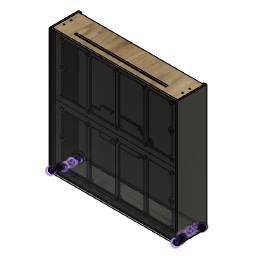
LEDMatrixCAD (Autodesk Fusion 360 design; units mm, degrees)
Autodesk Fusion 360 part; units mm, degrees
note: some values were not read from the file. Set by a fixed rule: which sketch regions a step uses.
sketch "PanelMount" plane through (0, 0, 0) normal (0, 1, 0) x (1, 0, 0)
  line L0 (0, 0) -> (256, 0)
  line L1 (256, 0) -> (256, -128)
  line L2 (256, -128) -> (0, -128)
  line L3 (0, -128) -> (0, 0)
  line L4 (128, -128) -> (128, 0) construction
  circle A0 centre (128, -116.25) radius 2.325
  circle A1 centre (128, -116.25) radius 6.975
  line L5 (0, -64) -> (256, -64) construction
  circle A2 centre (188, -116.25) radius 2.325
  circle A3 centre (188, -116.25) radius 6.975
  circle A4 centre (244, -116.25) radius 6.975
  circle A5 centre (244, -116.25) radius 2.325
  line L6 (244, -128) -> (244, 0) construction
  circle A6 centre (244, -64) radius 6.975
  circle A7 centre (244, -64) radius 2.325
  circle A8 centre (68, -116.25) radius 6.975
  circle A9 centre (68, -116.25) radius 2.325
  circle A10 centre (12, -116.25) radius 6.975
  circle A11 centre (12, -116.25) radius 2.325
  circle A12 centre (12, -64) radius 6.975
  circle A13 centre (12, -64) radius 2.325
  circle A14 centre (12, -11.75) radius 2.325
  circle A15 centre (12, -11.75) radius 6.975
  circle A16 centre (68, -11.75) radius 2.325
  circle A17 centre (68, -11.75) radius 6.975
  circle A18 centre (128, -11.75) radius 2.325
  circle A19 centre (128, -11.75) radius 6.975
  circle A20 centre (188, -11.75) radius 2.325
  circle A21 centre (188, -11.75) radius 6.975
  circle A22 centre (244, -11.75) radius 2.325
  circle A23 centre (244, -11.75) radius 6.975
  line L7 (12, -116.25) -> (244, -116.25)
  line L8 (244, -116.25) -> (244, -11.75)
  line L9 (244, -11.75) -> (12, -11.75)
  line L10 (12, -11.75) -> (12, -116.25)
  line L11 (0, -128) -> (-3, -128)
  line L12 (-3, -128) -> (-3, 0)
  line L13 (-3, 0) -> (0, 0)
  line L14 (256, -128) -> (259, -128)
  line L15 (259, -128) -> (259, 0)
  line L16 (259, 0) -> (256, 0)
  line L17 (65, -116.25) -> (65, -11.75)
  line L18 (71, -11.75) -> (71, -116.25)
  line L19 (68, -116.25) -> (68, -11.75) construction
  line L20 (125, -116.25) -> (125, -11.75)
  line L21 (131, -11.75) -> (131, -116.25)
  line L22 (131, -87.1298) -> (125, -87.1298) construction
  line L23 (65, -82.2396) -> (71, -82.2396) construction
  line L24 (185, -11.75) -> (185, -116.25)
  line L25 (191, -116.25) -> (191, -11.75)
  dimension "d301" = 4.65
  dimension "d302" = 4.65
  dimension "d305" = 60
  dimension "d306" = 116
  dimension "d308" = 256
  dimension "d309" = 128
  dimension "d310" = 11.75
  dimension "d348" = 3
  dimension "d429" = 6
  constraint horizontal L0
  constraint vertical L1
  constraint horizontal L2
  constraint vertical L3
  constraint coincident L0.start L3.end
  constraint midpoint L2 L4.start
  constraint midpoint L0 L4.end
  constraint coincident L4 A0.centre
  constraint concentric A0 A1
  constraint coincident L3 L5.start
  constraint coincident L1 L5.end
  constraint perpendicular L1 L5
  constraint midpoint L3 L5.start
  constraint concentric A2 A3
  constraint equal A1 A3
  constraint equal A0 A2
  constraint concentric A4 A5
  constraint equal A1 A4
  constraint equal A0 A5
  constraint coincident L2 L6.start
  constraint coincident L0 L6.end
  constraint perpendicular L0 L6
  constraint coincident A4.centre L6
  constraint concentric A6 A7
  constraint coincident L5 A6.centre
  constraint coincident L6 A6.centre
  constraint equal A1 A6
  constraint equal A0 A7
  constraint symmetric L4 A2 A9
  constraint symmetric L4 A3 A8
  constraint symmetric L4 A4 A10
  constraint symmetric L4 A5 A11
  constraint symmetric L4 A6 A12
  constraint symmetric L4 A7 A13
  constraint symmetric A0 L5 A18
  constraint symmetric A1 L5 A19
  constraint symmetric L5 A2 A20
  constraint symmetric L5 A3 A21
  constraint symmetric L5 A4 A23
  constraint symmetric L5 A5 A22
  constraint symmetric L5 A8 A17
  constraint symmetric L5 A9 A16
  constraint symmetric L5 A10 A15
  constraint symmetric L5 A11 A14
  constraint horizontal L7
  constraint vertical L8
  constraint horizontal L9
  constraint vertical L10
  constraint coincident A22.centre A23.centre
  constraint coincident A10.centre A11.centre
  constraint coincident A0.centre L7
  constraint coincident A2.centre L7
  constraint perpendicular L3 L11
  constraint perpendicular L11 L12
  constraint perpendicular L3 L13
  constraint perpendicular L1 L14
  constraint perpendicular L14 L15
  constraint perpendicular L1 L16
  constraint equal L11 L14
  constraint coincident L7 L17.start
  constraint coincident L9 L17.end
  constraint perpendicular L9 L17
  constraint coincident L9 L18.start
  constraint coincident L7 L18.end
  constraint perpendicular L7 L18
  constraint coincident A8.centre A9.centre
  constraint coincident A16.centre A17.centre
  constraint coincident L7 L20.start
  constraint coincident L9 L20.end
  constraint perpendicular L9 L20
  constraint coincident L9 L21.start
  constraint coincident L7 L21.end
  constraint perpendicular L7 L21
  constraint symmetric L4 L20 L21
  constraint coincident L21 L22.start
  constraint coincident L20 L22.end
  constraint perpendicular L20 L22
  constraint coincident L17 L23.start
  constraint coincident L18 L23.end
  constraint perpendicular L18 L23
  constraint equal L22 L23
  constraint symmetric L4 L17.start L25.start
  constraint symmetric L4 L17.end L25.end
  constraint symmetric L4 L18.start L24.start
  constraint symmetric L4 L18.end L24.end
  measures "d301" diameter of A0
  measures "d302" distance of A0 A1
  measures "d305" distance of A0.centre A2.centre
  measures "d306" distance of A0.centre A4.centre
  measures "d308" distance of L1.end L2.end
  measures "d309" distance of L0.start L2.end
  measures "d310" distance of L2 L7
  measures "d348" distance of L2.end L11.end
  measures "d429" distance of L17 L18
extrude "Extrude3" add sketch "PanelMount" against normal blind 3 contours L0 L1 L2 L3 | L3 L11 L12 L13 | L1 L14 L15 L16 | A0 A1 L7 | A0 A1 L7 L20 L21 | A1 L7 L21 | A1 L7 L20 | A1 A19 L20 L21 | A2 A3 L7 | A3 L7 L24 | A19 L9 L21 | A18 A19 L9 L20 L21 | A8 L7 L18 | A8 A9 L7 | A19 L9 L20 | A3 A21 L24 L25 | A2 A3 L7 L24 L25 | A3 L7 L25 | A18 A19 L9 | A8 A9 L7 L17 L18 | A8 A17 L17 L18 | A8 L7 L17 | A20 A21 L9 L24 L25 | A21 L9 L24 | A4 A5 L7 L8 | A4 A5 L7 L8 | A20 A21 L9 | A17 L9 L18 | A16 A17 L9 L17 L18 | A10 A11 L7 L10 | A10 A11 L7 L10 | A16 A17 L9 | A21 L9 L25 | A17 L9 L17 | A6 A7 L8 | A6 A7 L8 | A22 A23 L8 L9 | A22 A23 L8 L9 | A12 A13 L10 | A12 A13 L10 | A14 A15 L9 L10 | A14 A15 L9 L10 makes body 1
ref_plane "WorkPlane2" through (128, -1.5, 64) normal (1, 0, 0) x (0, 0, 1)
fillet "Fillet1" radius 1.5 12 edges at (9.8323, -3, 117.0908) (65.8323, -3, 117.0908) (125.8323, -3, 117.0908) (185.8323, -3, 117.0908) (241.8323, -3, 117.0908) (241.8323, -3, 64.8408) (241.8323, -3, 12.5908) (185.8323, -3, 12.5908) (125.8323, -3, 12.5908) (65.8323, -3, 12.5908) (9.8323, -3, 12.5908) (9.8323, -3, 64.8408) on bodies 1
pattern_linear "R-Pattern2" count 1 spacing 256 along (1, 0, 0) count 2 spacing 128 along (0, 0, 1) of bodies 1 makes body 2
sketch "Bracket" plane through (0, 0, 0) normal (0, 0, 1) x (1, 0, 0)
  line L0 (-6.65, -10.875) -> (-6.65, 51.475)
  line L1 (-6.65, 51.475) -> (-0.65, 51.475)
  line L2 (-0.65, -3.5) -> (-3.65, -3.5)
  line L3 (-3.65, -3.5) -> (-3.65, 0.5)
  line L4 (-3.65, 0.5) -> (-0.65, 0.5)
  line L5 (-0.65, 0) -> (-0.65, -3.5)
  line L6 (-0.65, 0.5) -> (-0.65, 0)
  line L7 (-0.65, -3.5) -> (-0.65, -7.5)
  line L8 (-0.65, -3) -> (-0.65, -3.5)
  line L9 (-0.65, 51.475) -> (-0.65, 0.5)
  line L10 (-0.65, 0) -> (-0.65, -3)
  line L11 (128, 11.7514) -> (128, -14.585) construction
  line L12 (-0.65, -7.5) -> (-3.65, -7.5)
  line L13 (-3.65, -7.5) -> (-3.65, -10.875)
  line L14 (-3.65, 0.5) -> (-3.65, 43.5)
  line L15 (-3.65, -3.5) -> (-3.65, -7.5)
  line L16 (-3, 0) -> (259, 0)
  line L17 (259, 0) -> (259, -3)
  line L18 (259, -3) -> (-3, -3)
  line L19 (-3, -3) -> (-3, 0)
  line L20 (-3.65, 43.5) -> (-0.65, 43.5)
  line L21 (-3.65, 43.5) -> (-3.65, 47.975)
  line L22 (-3.65, 47.975) -> (-0.65, 47.975)
  line L23 (-0.65, 38.5) -> (7.35, 38.5)
  line L24 (7.35, 38.5) -> (7.35, 43.5)
  line L25 (7.35, 43.5) -> (-0.65, 43.5)
  line L26 (-6.65, 18) -> (7.35, 18) construction
  line L27 (-0.65, 6.5) -> (7.35, 6.5)
  line L28 (7.35, 6.5) -> (7.35, 29.5)
  line L29 (7.35, 29.5) -> (-0.65, 29.5)
  circle A0 centre (3.35, 25.5) radius 1.5
  line L30 (3.35, 6.5) -> (3.35, 29.5) construction
  circle A1 centre (3.35, 10.5) radius 1.5
  line L31 (-3.65, -10.875) -> (-6.65, -10.875)
  line L32 (7.35, 43.5) -> (20, 43.5) construction
  line L33 (20, 43.5) -> (20, -7.5) construction
  line L34 (20, -7.5) -> (-0.65, -7.5) construction
  line L35 (20, 18) -> (7.35, 18) construction
  point P0 (128, 0)
  point P1 (128, 0)
  dimension "d334" = 4
  dimension "d335" = 3.375
  dimension "d349" = 0.65
  dimension "d350" = 0.5
  dimension "d351" = 0.5
  dimension "d353" = 3
  dimension "d354" = 3
  dimension "d356" = 43
  dimension "d359" = 4.475
  dimension "d360" = 3.5
  dimension "d361" = 8
  dimension "d362" = 5
  dimension "d366" = 8
  dimension "d376" = 3
  dimension "d379" = 4
  dimension "d452" = 23
  constraint vertical L9
  constraint perpendicular L1 L9
  constraint coincident L5.start L9
  constraint horizontal L2
  constraint vertical L3
  constraint horizontal L4
  constraint vertical L5
  constraint coincident L2.start L9
  constraint equal L6 L8
  constraint collinear L9 L10
  constraint perpendicular L12 L13
  constraint equal L2 L12
  constraint coincident L11 P1
  constraint coincident L9 L20.end
  constraint perpendicular L9 L20
  constraint perpendicular L20 L21
  constraint coincident L9 L22.end
  constraint perpendicular L9 L22
  constraint coincident L9 L23.start
  constraint perpendicular L9 L23
  constraint perpendicular L20 L24
  constraint perpendicular L9 L25
  constraint perpendicular L9 L26
  constraint coincident L9 L27.start
  constraint perpendicular L9 L27
  constraint perpendicular L27 L28
  constraint coincident L9 L29.end
  constraint perpendicular L9 L29
  constraint midpoint L28 L26.end
  constraint midpoint L27 L30.start
  constraint midpoint L29 L30.end
  constraint coincident A0.centre L30
  constraint symmetric L26 A0 A1
  constraint perpendicular L0 L31
  constraint coincident L0 L26.start
  constraint perpendicular L7 L12
  constraint perpendicular L24 L32
  constraint perpendicular L12 L33
  constraint perpendicular L7 L34
  constraint midpoint L33 L35.start
  constraint perpendicular L33 L35
  measures "d334" distance of L2 L12
  measures "d335" distance of L12.end L13.end
  measures "d349" distance of L3 L19
  measures "d350" distance of L2 L18
  measures "d351" distance of L4 L16
  measures "d353" distance of L9 L14
  measures "d354" distance of L0 L3
  measures "d356" distance of L4 L20
  measures "d359" distance of L20 L22
  measures "d360" distance of L1 L22
  measures "d361" distance of L9 L24
  measures "d362" distance of L23 L25
  measures "d366" distance of L27.start L27.end
  measures "d376" diameter of A0
  measures "d379" distance of L29 A0.centre
  measures "d452" distance of L27.end L28.end
extrude "Extrude4" add sketch "Bracket" along normal blind 256 separate body contours L0 L1 L3 L9 L13 L14 L15 L21 L22 L31 | L2 L7 L12 L15 | L4 L9 L14 L20 makes body 3
extrude "Extrude5" add sketch "Bracket" along normal blind 3.175 from surface at 256 contours L0 L1 L3 L9 L13 L14 L15 L21 L22 L31 bodies 3
extrude "Extrude6" add sketch "Bracket" against normal blind 3.175 contours L0 L1 L3 L9 L13 L14 L15 L21 L22 L31 bodies 3
extrude "Extrude7" add sketch "Bracket" along normal blind 8 contours L9 L23 L24 L25 bodies 3
extrude "Extrude8" add sketch "Bracket" along normal blind 3 contours L9 L27 L28 L29 bodies 3
sketch "MountTabHole" plane through (0, 43.5, 0) normal (0, 1, 0) x (-1, 0, 0)
  line L0 (-7.35, 0) -> (3.65, 0)
  line L1 (3.65, 0) -> (3.65, 256)
  line L2 (3.65, 256) -> (0.65, 256)
  line L3 (0.65, 256) -> (0.65, 8)
  line L4 (0.65, 8) -> (-7.35, 8)
  line L5 (-7.35, 8) -> (-7.35, 0)
  line L6 (0.65, 8) -> (0.65, 0)
  line L7 (-7.35, 8) -> (0.65, 0) construction
  line L8 (-7.35, 0) -> (0.65, 8) construction
  circle A0 centre (-3.35, 4) radius 1.5
  dimension "d383" = 3
  constraint coincident L3.end L4.start
  constraint coincident L0 L6.end
  constraint perpendicular L0 L6
  constraint coincident L4.end L5.start
  constraint coincident L0.start L5.end
  constraint midpoint L7 A0.centre
  measures "d383" diameter of A0
extrude "Extrude9" cut sketch "MountTabHole" against normal up to surface (5 mm away) contours A0 bodies 3
ref_plane "WorkPlane3" through (-3.65, 20.3, 128) normal (0, 0, 1) x (1, 0, 0)
mirror "Mirror5" about plane through (-3.65, 20.3, 128) normal (0, 0, 1) of "Extrude7", "Extrude8", "Extrude9"
mirror "Mirror2" about plane through (128, -1.5, 64) normal (1, 0, 0) of bodies 3 makes body 4
sketch "PiMount" plane through (0, 0, 0) normal (0, 1, 0) x (1, 0, 0)
  line L0 (128, -128) -> (128, 0)
  line L1 (166.5, -156.5) -> (89.5, -156.5)
  line L2 (85.5, -152.5) -> (85.5, -103.5)
  line L3 (89.5, -99.5) -> (166.5, -99.5)
  line L4 (170.5, -103.5) -> (170.5, -152.5)
  line L5 (166.5, -152.5) -> (108.5, -152.5) construction
  line L6 (108.5, -152.5) -> (108.5, -103.5) construction
  line L7 (108.5, -103.5) -> (166.5, -103.5) construction
  line L8 (166.5, -103.5) -> (166.5, -152.5) construction
  circle A0 centre (166.5, -152.5) radius 1.7
  circle A1 centre (108.5, -152.5) radius 1.7
  circle A2 centre (166.5, -103.5) radius 1.7
  circle A3 centre (108.5, -103.5) radius 1.7
  line L9 (166.5, -152.5) -> (166.5, -156.5) construction
  line L10 (166.5, -103.5) -> (166.5, -99.5) construction
  arc A4 (166.5, -156.5) -> (170.5, -152.5) centre (166.5, -152.5) ccw
  arc A5 (170.5, -103.5) -> (166.5, -99.5) centre (166.5, -103.5) ccw
  arc A6 (89.5, -99.5) -> (85.5, -103.5) centre (89.5, -103.5) ccw
  arc A7 (85.5, -152.5) -> (89.5, -156.5) centre (89.5, -152.5) ccw
  line L11 (128, -156.5) -> (128, -99.5) construction
  circle A8 centre (188, -116.25) radius 2.325
  circle A9 centre (188, -139.75) radius 2.325
  circle A10 centre (68, -139.75) radius 2.325
  circle A11 centre (68, -116.25) radius 2.325
  line L12 (172.5, -145.75) -> (190, -145.75)
  line L13 (194, -141.75) -> (194, -114.25)
  line L14 (190, -110.25) -> (172.5, -110.25)
  line L15 (256, -128) -> (0, -128)
  line L16 (188, -139.75) -> (188, -145.75) construction
  line L17 (188, -139.75) -> (194, -139.75) construction
  arc A12 (190, -145.75) -> (194, -141.75) centre (190, -141.75) ccw
  arc A13 (194, -114.25) -> (190, -110.25) centre (190, -114.25) ccw
  arc A14 (172.5, -145.75) -> (170.5, -147.75) centre (172.5, -147.75) ccw
  arc A15 (170.5, -108.25) -> (172.5, -110.25) centre (172.5, -108.25) ccw
  arc A16 (83.5, -110.25) -> (85.5, -108.25) centre (83.5, -108.25) ccw
  line L18 (66, -110.25) -> (83.5, -110.25)
  arc A17 (66, -110.25) -> (62, -114.25) centre (66, -114.25) ccw
  line L19 (62, -141.75) -> (62, -114.25)
  arc A18 (62, -141.75) -> (66, -145.75) centre (66, -141.75) ccw
  line L20 (83.5, -145.75) -> (66, -145.75)
  arc A19 (85.5, -147.75) -> (83.5, -145.75) centre (83.5, -147.75) ccw
  circle A20 centre (188, -139.75) radius 1.575
  circle A21 centre (188, -116.25) radius 1.575
  circle A22 centre (68, -139.75) radius 1.575
  circle A23 centre (68, -116.25) radius 1.575
  circle A24 centre (188, -139.75) radius 3.5
  point P0 (170.5, -156.5)
  point P1 (85.5, -156.5)
  dimension "d406" = 85
  dimension "d408" = 3.4
  dimension "d409" = 4
  dimension "d410" = 4
  dimension "d411" = 49
  dimension "d412" = 58
  dimension "d413" = 4
  dimension "d414" = 6
  dimension "d415" = 4
  dimension "d416" = 4
  dimension "d417" = 4
  dimension "d426" = 3.15
  dimension "d428" = 3.5
  constraint horizontal L1
  constraint vertical L2
  constraint horizontal L3
  constraint vertical L4
  constraint horizontal L5
  constraint vertical L6
  constraint horizontal L7
  constraint vertical L8
  constraint coincident L5.start L8.end
  constraint coincident L5.end L6.start
  constraint coincident L7.end L8.start
  constraint coincident L6.end L7.start
  constraint equal A0 A1
  constraint equal A0 A2
  constraint equal A0 A3
  constraint coincident L1 L9.end
  constraint perpendicular L1 L9
  constraint coincident L3 L10.end
  constraint perpendicular L3 L10
  constraint equal L9 L10
  constraint coincident P0 L1
  constraint coincident P0 L4
  constraint tangent L1 A4
  constraint tangent L4 A4
  constraint tangent L3 A5
  constraint tangent L4 A5
  constraint equal A4 A5
  constraint tangent L2 A6
  constraint tangent L3 A6
  constraint equal A4 A6
  constraint coincident P1 L1
  constraint coincident P1 L2
  constraint tangent L1 A7
  constraint tangent L2 A7
  constraint equal A4 A7
  constraint midpoint L1 L11.start
  constraint midpoint L3 L11.end
  constraint coincident L0 L11.end
  constraint perpendicular L4 L12
  constraint perpendicular L12 L13
  constraint perpendicular L4 L14
  constraint symmetric L12 L14 L15
  constraint coincident A9.centre L16.start
  constraint coincident L12 L16.end
  constraint perpendicular L12 L16
  constraint coincident L13 L17.end
  constraint perpendicular L13 L17
  constraint equal L16 L17
  constraint tangent L12 A12
  constraint tangent L13 A12
  constraint tangent L13 A13
  constraint tangent L14 A13
  constraint equal A12 A13
  constraint tangent L4 A14
  constraint tangent L12 A14
  constraint coincident L4 A14.end
  constraint tangent L14 A15
  constraint tangent L4 A15
  constraint coincident L4 A15.start
  constraint symmetric L11 L12.end A18.end
  constraint symmetric L11 L13.start L19.start
  constraint symmetric L11 A12 A18
  constraint symmetric L11 L13.end A17.end
  constraint symmetric L11 L14.start L18.start
  constraint symmetric L11 A13 A17
  constraint symmetric L11 A14.end A19.start
  constraint symmetric L11 L12.start L20.start
  constraint symmetric L11 A14 A19
  constraint symmetric L11 L14.end A16.start
  constraint symmetric L11 A15.start A16.end
  constraint symmetric L11 A15 A16
  constraint symmetric L1 L3 L15
  constraint concentric A9 A20
  constraint concentric A8 A21
  constraint equal A20 A21
  constraint symmetric L11 A20 A22
  constraint symmetric L11 A21 A23
  constraint concentric A9 A24
  measures "d406" distance of P0 P1
  measures "d408" diameter of A0
  measures "d409" distance of L1 L5.start
  measures "d410" distance of L4 L5.start
  measures "d411" distance of L5.start L7.end
  measures "d412" distance of L5.start L5.end
  measures "d413" radius of A4
  measures "d414" distance of A9.centre L12
  measures "d415" radius of A12
  measures "d416" diameter of A14
  measures "d417" diameter of A15
  measures "d426" diameter of A20
  measures "d428" radius of A24
extrude "Extrude10" add sketch "PiMount" along normal blind 3 from surface at 4.3 separate body contours L0 L2 L3 A6 L15 | L0 L3 L4 A5 L15 | L1 L2 L4 A4 A7 L15 | L4 L12 L13 L15 A12 A14 | L4 L13 L14 L15 A13 A15 | L2 L15 A16 L18 A17 L19 | L2 L15 L19 A18 L20 A19 | A8 | A9 | A10 | A11 | A24 makes body 5
extrude "Extrude11" add sketch "PiMount" along normal up to surface (4.3 mm away) separate body contours A24 makes body 6
sketch "Bottom/Top Cover" plane through (0, 0, 0) normal (0, 0, 1) x (1, 0, 0)
  line L0 (-3.65, -7.5) -> (-3.65, -3.5)
  line L1 (-3.65, -3.5) -> (-0.65, -3.5)
  line L2 (-0.65, -3.5) -> (-0.65, -7.5)
  line L3 (-0.65, -7.5) -> (-3.65, -7.5)
  circle A0 centre (3.35, 25.5) radius 1.5
  circle A1 centre (3.35, 10.5) radius 1.5
  line L4 (-3.65, 0.5) -> (-3.65, 43.5)
  line L5 (-3.65, 43.5) -> (7.35, 43.5)
  line L6 (7.35, 43.5) -> (7.35, 38.5)
  line L7 (7.35, 38.5) -> (-0.65, 38.5)
  line L8 (-0.65, 38.5) -> (-0.65, 29.5)
  line L9 (-0.65, 29.5) -> (7.35, 29.5)
  line L10 (7.35, 29.5) -> (7.35, 6.5)
  line L11 (7.35, 6.5) -> (-0.65, 6.5)
  line L12 (-0.65, 6.5) -> (-0.65, 0.5)
  line L13 (-0.65, 0.5) -> (-3.65, 0.5)
  circle A2 centre (252.65, 25.5) radius 1.5
  circle A3 centre (252.65, 10.5) radius 1.5
  line L14 (259.65, 43.5) -> (259.65, 0.5)
  line L15 (259.65, 0.5) -> (256.65, 0.5)
  line L16 (256.65, 0.5) -> (256.65, 6.5)
  line L17 (256.65, 6.5) -> (248.65, 6.5)
  line L18 (248.65, 6.5) -> (248.65, 29.5)
  line L19 (248.65, 29.5) -> (256.65, 29.5)
  line L20 (256.65, 29.5) -> (256.65, 38.5)
  line L21 (256.65, 38.5) -> (248.65, 38.5)
  line L22 (248.65, 38.5) -> (248.65, 43.5)
  line L23 (248.65, 43.5) -> (259.65, 43.5)
  line L24 (259.65, -3.5) -> (259.65, -7.5)
  line L25 (259.65, -7.5) -> (256.65, -7.5)
  line L26 (256.65, -7.5) -> (256.65, -3.5)
  line L27 (256.65, -3.5) -> (259.65, -3.5)
  line L28 (259.65, 43.5) -> (-3.65, 43.5) construction
  line L29 (-3.65, 43.5) -> (-3.65, -7.5)
  line L30 (259.65, -7.5) -> (-3.65, -7.5)
  line L31 (259.65, -7.5) -> (259.65, 43.5)
  line L32 (259.65, 47.975) -> (259.65, -10.875)
  line L33 (-3.65, 47.975) -> (-3.65, -10.875)
  line L34 (256.65, 47.975) -> (259.65, 47.975)
  line L35 (-0.65, 47.975) -> (-3.65, 47.975)
  line L36 (-0.65, 47.975) -> (256.65, 47.975)
  line L37 (-0.65, 0.5) -> (256.65, 0.5) construction
  line L38 (-0.65, 3.5) -> (256.65, 3.5)
  line L39 (256.65, 8.5) -> (-0.65, 8.5)
  line L40 (128, 3.5) -> (128, 8.5) construction
  line L41 (32, 3.5) -> (32, 8.5)
  line L42 (224, 3.5) -> (224, 8.5)
  line L43 (-0.65, 6.5) -> (-0.65, 8.5) construction
  line L44 (256.65, 6.5) -> (256.65, 8.5) construction
  dimension "d445" = 3
  dimension "d446" = 5
  dimension "d447" = 192
  constraint coincident L14.start L23.end
  constraint coincident L4.end L5.start
  constraint coincident L0.start L3.end
  constraint coincident L24.end L25.start
  constraint coincident L35.start L36.start
  constraint coincident L34.start L36.end
  constraint coincident L12.end L13.start
  constraint coincident L15.end L16.start
  constraint coincident L12 L38.start
  constraint coincident L16 L38.end
  constraint perpendicular L16 L38
  constraint coincident L16 L39.start
  constraint coincident L12 L39.end
  constraint perpendicular L12 L39
  constraint midpoint L38 L40.start
  constraint midpoint L39 L40.end
  constraint coincident L38 L41.start
  constraint coincident L39 L41.end
  constraint perpendicular L39 L41
  constraint coincident L38 L42.start
  constraint coincident L39 L42.end
  constraint perpendicular L39 L42
  constraint symmetric L40 L41 L42
  constraint coincident L11.end L12.start
  constraint coincident L16.end L17.start
  measures "d445" distance of L37 L38
  measures "d446" distance of L38 L39
  measures "d447" distance of L41 L42
extrude "Extrude12" add sketch "Bracket" sketch "Bottom/Top Cover" along normal up to surface separate body contours L4 L9 L14 L20 | L9 L27 L28 L29 of sketch 2 contours L0 L1 L2 L3 L29 L30 L33 | L1 L2 L12 L13 L15 L16 L26 L27 L29 L30 L31 L32 L33 L38 | L4 L5 L6 L7 L8 L9 L10 L11 L12 L13 L29 L33 | L24 L25 L26 L27 L30 L31 L32 | L5 L6 L7 L8 L9 L10 L18 L19 L20 L21 L22 L23 L32 L33 L34 L35 L36 L39 | L10 L11 L12 L38 L39 L41 | L14 L15 L16 L17 L18 L19 L20 L21 L22 L23 L31 L32 | L16 L17 L18 L38 L39 L42 end surface through (0, 0, -3.175) normal (0, 0, -1) offset 0 makes body 7
mirror "Mirror6" about plane through (-3.65, 20.3, 128) normal (0, 0, 1) of bodies 7 makes body 8
sketch "BackPlate" plane through (0, 43.5, 0) normal (0, 1, 0) x (-1, 0, 0)
  line L0 (-7.35, 0) -> (3.65, 0)
  line L1 (3.65, 256) -> (-7.35, 256)
  line L2 (-259, 128) -> (-259, 0)
  line L3 (3, 128) -> (3, 0)
  line L4 (-259, 0) -> (3, 0)
  line L5 (-259, 256) -> (3, 256)
  line L6 (-259, 0) -> (-259, 256)
  line L7 (-254.15, -3.175) -> (-251.15, -3.175)
  line L8 (-254.15, -3.175) -> (-251.15, -3.175)
  line L9 (-4.85, -3.175) -> (-1.85, -3.175)
  line L10 (-4.85, -3.175) -> (-1.85, -3.175)
  line L11 (-254.15, 259.175) -> (-251.15, 259.175)
  line L12 (-254.15, 259.175) -> (-251.15, 259.175)
  line L13 (-4.85, 259.175) -> (-1.85, 259.175)
  line L14 (-4.85, 259.175) -> (-1.85, 259.175)
  line L15 (3, 0) -> (3, -3.175)
  line L16 (-259, 0) -> (-259, -3.175)
  line L17 (-259, 256) -> (-259, 259.175)
  line L18 (3, 256) -> (3, 128)
  line L19 (3, 256) -> (3, 259.175)
  circle A0 centre (-225, 20) radius 7.0711
  line L20 (3.65, -3.175) -> (-259.65, -3.175)
  line L21 (-259.65, 259.175) -> (3.65, 259.175)
  line L22 (-32, -3.175) -> (-224, -3.175)
  line L23 (-224, -3.175) -> (-32, -3.175)
  line L24 (-32, 259.175) -> (-224, 259.175)
  line L25 (-224, 259.175) -> (-32, 259.175)
  line L26 (-259.65, -3.175) -> (3.65, -3.175)
  line L27 (3.65, 259.175) -> (-259.65, 259.175)
  dimension "d436" = 256
  constraint coincident L2.end L4.start
  constraint perpendicular L5 L6
  constraint coincident L3.end L4.end
  constraint coincident L5.end L18.start
  measures "d436" distance of L4 L5
extrude "Extrude14" add sketch "BackPlate" along normal blind 3.175 from surface at 0.65 separate body contours L0 L1 L2 L3 L4 L5 L6 L18 makes body 9
sketch "Sketch20" plane through (0, -10.875, 0) normal (0, -1, 0) x (1, 0, 0)
  line L0 (-3.65, -3.175) -> (-3.65, 259.175)
  line L1 (-3.65, 259.175) -> (-6.65, 259.175)
  line L2 (-6.65, 259.175) -> (-6.65, -3.175)
  line L3 (-6.65, -3.175) -> (-3.65, -3.175)
  line L4 (259.65, 259.175) -> (259.65, -3.175)
  line L5 (259.65, -3.175) -> (262.65, -3.175)
  line L6 (262.65, -3.175) -> (262.65, 259.175)
  line L7 (262.65, 259.175) -> (259.65, 259.175)
  line L8 (-3.65, 259.175) -> (259.65, 259.175)
  line L9 (259.65, -3.175) -> (-3.65, -3.175)
  constraint coincident L0.end L1.start
  constraint coincident L4.start L7.end
  constraint coincident L4.end L5.start
  constraint coincident L0.start L3.end
extrude "Extrude15" add sketch "Sketch20" against normal blind 3.375 separate body contours L0 L4 L8 L9 makes body 10
equation "PanelWidth = 256 mm"
equation "PanelHeight = 128 mm"
equation "XPanels = 1"
equation "YPanels = 2"
equation "MountThickness = 3 mm"
equation "PanelStudDia = 4 mm"
equation "HorizonalMountingTabSideLen = 10 mm"
equation "StudRingPadding = 7 mm" comment "Defines space between stud hole and outer ring (similar to a radius, so a value of 4 will add 8mm to original diameter)"
equation "TightFitTolerance = 0.2 mm"
equation "JoiningScrewSize = 4 mm"
equation "LooseFitTolerance = 0.65 mm"
equation "d301 = PanelStudDia + LooseFitTolerance"
equation "d302 = PanelStudDia + LooseFitTolerance"
equation "d308 = PanelWidth"
equation "d309 = PanelHeight"
equation "d311 = -MountThickness"
equation "d317 = XPanels"
equation "d318 = YPanels"
equation "d319 = PanelWidth"
equation "d320 = -PanelHeight"
equation "d332 = PanelHeight * YPanels"
equation "d334 = 2 mm + 2 mm" comment "Measured 5.31mm from panel to outside acryllic edge. (5.31mm - 1/8\" ~= 2mm). Edit: had to add 2mm for extra space"
equation "d335 = 3.175 mm + TightFitTolerance"
equation "d348 = SlotDepth"
equation "d349 = LooseFitTolerance"
equation "SlotDepth = 3 mm"
equation "d353 = SlotDepth"
equation "AcrylicThickness = ( 1 / 8 ) * 1 in"
equation "BackplateThickness = ( 1 / 8 ) * 1 in"
equation "d359 = BackplateThickness + LooseFitTolerance * 2"
equation "d361 = ScrewTabSideLength"
equation "d363 = ScrewTabSideLength"
equation "ScrewTabSideLength = 8 mm"
equation "d366 = ScrewTabSideLength"
equation "d368 = MountThickness"
equation "ScrewDiameter = 3 mm"
equation "d376 = ScrewDiameter"
equation "d379 = ScrewTabSideLength / 2"
equation "d383 = ScrewDiameter"
equation "d408 = 2.75 mm + LooseFitTolerance"
equation "d419 = MountThickness"
equation "PanelStudScrewDia = 2.5 mm"
equation "d426 = PanelStudScrewDia + LooseFitTolerance"
equation "d436 = YPanels * PanelHeight"
equation "d437 = LooseFitTolerance"
equation "d447 = PanelWidth * XPanels * 0.75"
named bodies: "BottomScreenPanel", "TopScreenPanel", "LeftBracket", "RightBracket", "PiMount", "PiMountSpacer", "Bottomplate", "Topplate", "Backplate", "FrontPanel"
